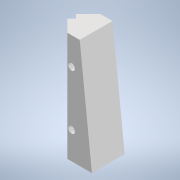
# Autodesk Inventor part: tower
Saved by Autodesk Inventor 2022 (Build 260153000, 153)
## iProperties
Created: 2022-04-10
Part Number: tower
Material: Generic
Document SubType Name: Modeling
Designer: Cody
Density: 1 g/cm^3
Appearance: Default
Author: Cody
Autodesk Inventor part; units mm, degrees
ref_plane "YZ Plane" through (0, 0, 0) normal (1, 0, 0) x (0, 1, 0)
ref_plane "XZ Plane" through (0, 0, 0) normal (0, 1, 0) x (-1, 0, 0)
ref_plane "XY Plane" through (0, 0, 0) normal (0, 0, 1) x (1, 0, 0)
sketch "Sketch2" plane through (0, 0, 0) normal (0, 0, 1) x (1, 0, 0)
  line L0 (0, 0) -> (0, 100)
  line L1 (0, 100) -> (25, 100)
  line L2 (25, 100) -> (42.6378, -0.0289)
  line L3 (0, 0) -> (43.61, 0)
  point P0 (42.6327, 0)
  dimension "d0" = 100
  dimension "d1" = 25
  dimension "d2" = 100
  constraints: 8 end point, 1 horizontal, 1 perpendicular, 1 vertical
  measures "d0" distance of L0.start L0.end
  measures "d1" distance of L0.end L1.end
  measures "d2" angle of L1 L2
extrude "Extrusion1" add sketch "Sketch2" along normal blind 30
sketch "Sketch3" plane through (0, 0, 0) normal (0, -1, 0) x (1, 0, 0)
  line L0 (25, 0) -> (25, 30) construction
  circle A0 centre (25, 15) radius 3
  line L1 (0, 0) -> (0, 30) projected
  line L2 (0, 0) -> (53.0924, 0) construction
  line L3 (0, 30) -> (48.2288, 30) construction
  line L4 (0, 0) -> (42.6327, 0) projected
  line L5 (0, 0) -> (0, 2)
  line L6 (0, 2) -> (43.5551, 45.5551)
  line L7 (0, 30) -> (42.6327, 30) projected
  line L8 (0, 30) -> (0, 28)
  line L9 (0, 28) -> (39.6669, -11.6669)
  point P0 (13, 15)
  dimension "d6" = 6
  dimension "d8" = 25
  dimension "d11" = 2
  dimension "d12" = 135
  dimension "d13" = 2
  dimension "d14" = 135
  constraints: 14 end point, 2 horizontal, 2 point on line, 1 centre point, 1 midpoint
  measures "d6" diameter of A0
  measures "d8" distance from line of L1 L0.start
  measures "d11" distance of L1.start L5.end
  measures "d12" angle of L5 L6
  measures "d13" distance of L1.end L8.end
  measures "d14" angle of L9 L8
extrude "Extrusion2" cut sketch "Sketch3" against normal up to surface (100 mm away) contours L1 L9 L6
hole "Hole1" at (25, 0, 15) direction (0, 1, 0) diameter 5.9175 depth 20 tip angle 118 thread size "M7x1" class "6H" standard "ANSI Metric M Profile"
sketch "Sketch4" plane through (0, 100, 0) normal (0, 1, 0) x (1, 0, 0)
  line L0 (0, -31) -> (25, -31)
  line L1 (25, -31) -> (25, -30)
  line L2 (42.6327, -30) -> (25, -30) projected
  line L3 (0, -30) -> (42.6327, -30) projected
  line L4 (25, -30) -> (0, -30)
  line L5 (0, -28) -> (13, -15) projected
  line L6 (0, -30) -> (0, -28)
  line L7 (13, -15) -> (0, -2) projected
  line L8 (0, -28) -> (13, -15)
  line L9 (13, -15) -> (0, -2)
  line L10 (0, -2) -> (0, 0)
  line L11 (0, 0) -> (25, 0)
  line L12 (0, 0) -> (42.6327, 0) projected
  line L13 (25, 0) -> (25, 1)
  line L14 (25, 1) -> (0, 1)
  line L15 (0, 1) -> (-1, 1)
  line L16 (-1, 1) -> (-1, -2)
  line L17 (-1, -2) -> (12, -15)
  line L18 (12, -15) -> (-1, -28)
  line L19 (-1, -28) -> (-1, -31)
  line L20 (-1, -31) -> (0, -31)
  dimension "d25" = 1
  dimension "d26" = 1
  dimension "d27" = 1
  constraints: 32 end point, 7 perpendicular, 5 point on line, 4 equal length, 1 horizontal
  measures "d25" distance of L3.start L0.start
  measures "d26" distance of L11.end L13.end
  measures "d27" distance of L14.end L15.end
sketch "Sketch5" plane through (0, 0, 0) normal (0, 0, -1) x (-1, 0, 0)
  line L0 (-25, 100) -> (0, 100) projected
  line L1 (0, 100) -> (0, 75)
  line L2 (0, 100) -> (0, 0) projected
  line L3 (0, 75) -> (-24, 75)
  line L4 (0, 0) -> (0, 25)
  line L5 (0, 25) -> (-24, 25)
  circle A0 centre (-24, 25) radius 3
  circle A1 centre (-24, 75) radius 3
  dimension "d28" = 25
  dimension "d29" = 24
  dimension "d30" = 25
  dimension "d31" = 24
  dimension "d32" = 6
  dimension "d33" = 6
  constraints: 8 end point, 2 centre point, 2 coincident, 2 perpendicular, 2 point on line
  measures "d28" distance of L0.end L1.end
  measures "d29" distance of L1.end L3.end
  measures "d30" distance of L2.end L4.end
  measures "d31" distance of L4.end L5.end
  measures "d32" diameter of A0
  measures "d33" diameter of A1
extrude "Extrusion3" cut sketch "Sketch5" against normal up to surface (30 mm away)
sketch "Sketch6" plane through (0, 100, 0) normal (0, 1, 0) x (1, 0, 0)
  line L0 (13, -15) -> (9.1109, -11.1109)
  line L1 (13, -15) -> (0, -2) projected
  line L2 (9.1109, -11.1109) -> (20.2218, 0)
  line L3 (13, -15) -> (0, -28) projected
  line L4 (13, -15) -> (9.1109, -18.8891)
  line L5 (9.1109, -18.8891) -> (20.2218, -30)
  line L6 (25, -30) -> (0, -30) projected
  line L7 (20.2218, -30) -> (0, -30)
  line L8 (0, -30) -> (0, -28)
  line L9 (0, -28) -> (9.1109, -18.8891)
  line L10 (0, -2) -> (13, -15) projected
  line L11 (9.1109, -11.1109) -> (0, -2)
  line L12 (0, -2) -> (0, 0)
  line L13 (0, 0) -> (20.2218, 0)
  line L14 (25, 0) -> (0, 0) projected
  line L15 (13, -15) -> (9.1109, -18.8891)
  dimension "d36" = 5.5
  dimension "d44" = 5.5
  constraints: 23 end point, 4 collinear, 3 perpendicular, 3 point on line
  measures "d36" distance of L0.start L0.end
  measures "d44" distance of L0.start L4.end
extrude "Extrusion4" cut sketch "Sketch6" against normal up to next
sketch "Sketch7" plane through (25, 100, 30) normal (0, 1, 0) x (1, 0, 0)
  line L0 (17.6327, 0) -> (0, 0) projected
  line L1 (17.6327, 30) -> (0, 30) projected
  line L2 (0, 0) -> (17.6327, 0)
  line L3 (17.6327, 0) -> (17.6327, 30)
  line L4 (17.6327, 30) -> (0, 30)
  line L5 (0, 30) -> (0, 0)
  point P0 (-25, 30)
  constraints: 8 end point, 2 parallel, 1 horizontal, 1 perpendicular
extrude "Extrusion5" add sketch "Sketch7" along normal up to surface surface through (42.6327, 0, 0) normal (0.9848078, 0.1736482, 0)
sketch "Sketch8" plane through (0, 0, 0) normal (0, 0, -1) x (-1, 0, 0)
  line L0 (-42.6327, 100) -> (-42.6327, 0) projected
  line L1 (-42.6327, 100) -> (-20.2218, 100) projected
  line L2 (-42.6327, 100) -> (-20.2218, 100)
  line L3 (-20.2218, 100) -> (-31.4273, 100)
  line L4 (-20.2218, 0) -> (-42.6327, 0) projected
  line L5 (-31.4273, 100) -> (-42.6327, 0)
  point P0 (0, 0)
  constraints: 6 end point, 1 collinear, 1 midpoint
extrude "Extrusion6" cut sketch "Sketch8" against normal up to next
sketch "Sketch10" plane through (0, 0, 0) normal (0, 0, -1) x (-1, 0, 0)
  line L0 (-20.2218, 100) -> (-9.1109, 100) projected
  line L1 (-20.2218, 100) -> (-24, 78)
  circle A0 centre (-24, 75) radius 3 projected
  line L2 (-24, 72) -> (-24, 28)
  circle A1 centre (-24, 25) radius 3 projected
  circle A2 centre (-24, 75) radius 3
  circle A3 centre (-24, 25) radius 3
  point P0 (0, 0)
  constraints: 4 end point, 2 centre point, 2 coincident, 2 point on circle, 1 concentric, 1 vertical, 1 vertical alignment, 2 other
ref_plane "Work Plane2" through (0, 0, -1) normal (0, 0, -1) x (-1, 0, 0)
sketch "Sketch11" plane through (0, 0, -1) normal (0, 0, -1) x (-1, 0, 0)
  line L0 (-20.2218, 0) -> (-20.2218, 100) projected
  line L1 (-20.2218, 100) -> (-24, 78)
  circle A0 centre (-24, 75) radius 3 projected
  circle A1 centre (-24, 75) radius 3
  line L2 (-24, 72) -> (-24, 28)
  circle A2 centre (-24, 25) radius 3 projected
  circle A3 centre (-24, 25) radius 3
  point P0 (0, 0)
  constraints: 4 end point, 3 vertical alignment, 2 coincident, 1 centre point, 1 vertical, 5 other
body "Solid1"
